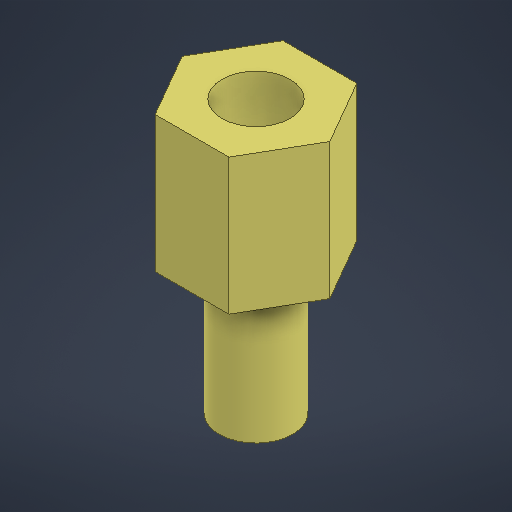
# Autodesk Inventor part: distances
Saved by Autodesk Inventor 2026.2 (Build 302298000, 298)
## iProperties
Created: 2026-02-13
Part Number: distances
Material: Generic
Document SubType Name: Modeling
Designer: test
Density: 1 g/cm^3
Appearance: Default
Author: test
Autodesk Inventor part; units mm, degrees
ref_plane "YZ Plane" through (0, 0, 0) normal (1, 0, 0) x (0, 1, 0)
ref_plane "XZ Plane" through (0, 0, 0) normal (0, 1, 0) x (-1, 0, 0)
ref_plane "XY Plane" through (0, 0, 0) normal (0, 0, 1) x (1, 0, 0)
sketch "Sketch1" plane through (0, 0, 0) normal (0, 1, 0) x (-1, 0, 0)
  line L0 (-1.3568, -2.35) -> (-2.7135, 0)
  line L1 (-2.7135, 0) -> (-1.3568, 2.35)
  line L2 (-1.3568, 2.35) -> (1.3568, 2.35)
  line L3 (1.3568, 2.35) -> (2.7135, 0)
  line L4 (2.7135, 0) -> (1.3568, -2.35)
  line L5 (1.3568, -2.35) -> (-1.3568, -2.35)
  point P0 (0, 0)
  point P1 (0, 0)
  dimension "d13" = 4.7
  constraints: 12 end point, 13 other
  measures "d13" distance between parallel lines of L3 L0
extrude "Extrusion1" add sketch "Sketch1" along normal blind 5
sketch "Sketch3" plane through (0, 0, 0) normal (0, -1, 0) x (1, 0, 0)
  circle A0 centre (0, 0) radius 1.35
  dimension "d12" = 2.7
  constraints: 1 centre point, 1 coincident
  measures "d12" diameter of A0
extrude "Extrusion2" add sketch "Sketch3" along normal blind 5
sketch "Sketch6" plane through (0, 5, 0) normal (0, 1, 0) x (1, 0, 0)
  point P0 (0, 0)
  point P1 (0, 0)
  constraints: 1 coincident
hole "Hole1" at (0, 5, 0) direction (0, -1, 0) diameter 2.5 depth 4 tip angle 118
body "Solid1"
